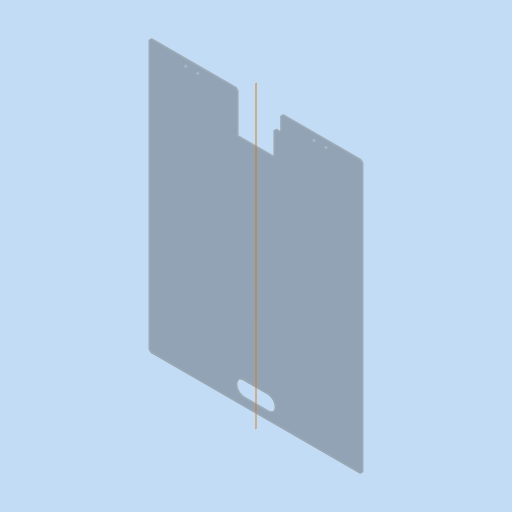
# Autodesk Inventor part: enc-BottomPanel
Saved by Autodesk Inventor 2023.2 (Build 272271000, 271)
## iProperties
Created: 2023-12-04
Part Number: enc-BottomPanel
Material: Generisch
Document SubType Name: Modeling
Designer: Nils Bade
Density: 1 g/cm^3
Appearance: PVC Verglasung
Author: Nils Bade
Autodesk Inventor part; units mm, degrees
ref_plane "XZ Plane" through (0, 0, 0) normal (0, 1, 0) x (-1, 0, 0)
ref_plane "XY Plane" through (0, 0, 0) normal (0, 0, 1) x (1, 0, 0)
sketch "Skizze1" plane through (0, 0, 0) normal (0, 0, 1) x (1, 0, 0)
  line L0 (-267, 340) -> (267, 340)
  line L1 (267, 340) -> (267, -340)
  line L2 (267, -340) -> (-267, -340)
  line L3 (-267, -340) -> (-267, 340)
  line L4 (-267, 340) -> (267, -340) construction
  line L5 (267, 340) -> (-267, -340) construction
  line L6 (-45, 340) -> (45, 340)
  line L7 (45, 340) -> (45, 238)
  line L8 (45, 238) -> (-45, 238)
  line L9 (-45, 238) -> (-45, 340)
  line L10 (0, 476) -> (0, -476) construction
  line L11 (0, 340) -> (62, 340)
  line L12 (62, 340) -> (62, 300)
  line L13 (62, 300) -> (0, 300)
  line L14 (0, 300) -> (0, 340)
  line L15 (-267, 323) -> (267, 323) construction
  circle A0 centre (-175.2, 323) radius 3.25
  line L16 (-160.2, 340) -> (-160.2, -340) construction
  circle A1 centre (-145.2, 323) radius 3.25
  circle A2 centre (175.2, 323) radius 3.25
  circle A3 centre (145.2, 323) radius 3.25
  line L17 (-30, -302) -> (30, -302) construction
  line L18 (-30, -320) -> (30, -320)
  line L19 (30, -284) -> (-30, -284)
  arc A4 (-30, -284) -> (-30, -320) centre (-30, -302) ccw
  arc A5 (30, -320) -> (30, -284) centre (30, -302) ccw
  point P0 (0, 0)
  point P1 (0, 238)
  point P2 (45, 300)
  point P3 (0, -302)
  dimension "d0" = 534
  dimension "d1" = 102
  dimension "d3" = 62
  dimension "d4" = 45
  dimension "d5" = 17
  dimension "d6" = 6.5
  dimension "d7" = 680
  dimension "d8" = 40
  dimension "d9" = 106.8
  dimension "d10" = 15
  dimension "d16" = 60
  dimension "d17" = 18
  dimension "d18" = 20
  constraints: 40 end point, 9 point on line, 7 parallel, 6 centre point, 6 perpendicular, 5 midpoint, 4 point on circle, 4 tangent, 3 horizontal, 3 symmetric about line, 3 other
  measures "d0" distance of L1.end L2.end
  measures "d1" distance between parallel lines of L0 L8
  measures "d3" distance between parallel lines of L10 L12
  measures "d4" distance between parallel lines of L9 L10
  measures "d5" distance between parallel lines of L0 L15
  measures "d6" diameter of A0
  measures "d7" distance of L0.end L1.end
  measures "d8" distance between parallel lines of L0 L13
  measures "d9" distance between parallel lines of L3 L16
  measures "d10" distance from line of L16 A0.centre
  measures "d16" distance of L17.start L17.end
  measures "d17" radius of A5
  measures "d18" distance between parallel lines of L2 L18
extrude "Extrusion1" add sketch "Skizze1" along normal blind 3 contours L0 L9 L8 L7 L13 L12 L1 L2 L3
chamfer "Fase1" distance 5 angle 45 7 edges at (-45, 340, 1.5) (45, 300, 1.5) (62, 340, 1.5) (267, 340, 1.5) (-267, 340, 1.5) (-267, -340, 1.5) (267, -340, 1.5)
equation "\"d9\" = 0.2 * d0"
